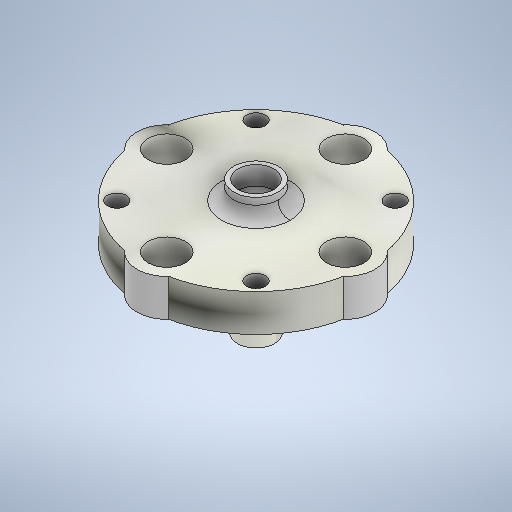
# Autodesk Inventor part: Redesign_Spinner
Saved by Autodesk Inventor 2025.1 (Build 291241000, 241)
## iProperties
Created: 2024-12-23
Part Number: Redesign_Spinner
Material: Generic
Document SubType Name: Modeling
Designer: m_kni
Density: 1 g/cm^3
Appearance: Default
Author: m_kni
Autodesk Inventor part; units mm, degrees
ref_plane "YZ Plane" through (0, 0, 0) normal (1, 0, 0) x (0, 1, 0)
ref_plane "XZ Plane" through (0, 0, 0) normal (0, 1, 0) x (-1, 0, 0)
ref_plane "XY Plane" through (0, 0, 0) normal (0, 0, 1) x (1, 0, 0)
sketch "Sketch1" plane through (0, 0, 0) normal (0, 1, 0) x (-1, 0, 0)
  circle A0 centre (0, 0) radius 2.5
  dimension "d0" = 5
  constraints: 1 centre point, 1 coincident
  measures "d0" diameter of A0
extrude "Extrusion1" add sketch "Sketch1" along normal blind 10.4
sketch "Sketch2" plane through (0, 10.4, 0) normal (0, 1, 0) x (1, 0, 0)
  circle A0 centre (0, 0) radius 12
  circle A1 centre (-12, 0) radius 1.5
  circle A2 centre (-12, 0) radius 2.5
  circle A3 centre (0, -12) radius 1.5
  circle A4 centre (0, -12) radius 2.5
  circle A5 centre (12, 0) radius 1.5
  circle A6 centre (12, 0) radius 2.5
  circle A7 centre (0, 12) radius 1.5
  circle A8 centre (0, 12) radius 2.5
  circle A9 centre (0, 0) radius 14.9832
  circle A10 centre (12, 0) radius 4
  circle A11 centre (0, -12) radius 4
  circle A12 centre (-12, 0) radius 4
  circle A13 centre (0, 12) radius 4
  point P0 (2.9628, -14.6873)
  point P1 (-2.9628, -14.6873)
  point P2 (-14.6873, -2.9628)
  point P3 (-14.6873, 2.9628)
  point P4 (-2.9628, 14.6873)
  point P5 (2.9628, 14.6873)
  point P6 (14.6873, 2.9628)
  point P7 (14.6873, -2.9628)
  dimension "d3" = 24
  dimension "d4" = 3
  dimension "d5" = 5
  dimension "d8" = 360
  dimension "d22" = 8
  dimension "d23" = 8
  dimension "d24" = 8
  dimension "d25" = 8
  constraints: 14 centre point, 6 coincident, 2 point on circle, 17 other
  measures "d3" diameter of A0
  measures "d4" diameter of A1
  measures "d5" diameter of A2
  measures "d22" diameter of A10
  measures "d23" diameter of A11
  measures "d24" diameter of A12
  measures "d25" diameter of A13
extrude "Extrusion2" add sketch "Sketch2" along normal blind 5 contours A6 A0 A10 | A0 A10 A9 A6 | A10 A0 A11 A12 A13 | A0 A13 A9 A10 | A10 A9 A11 A0 | A13 A0 A8 | A0 A8 A13 A9 | A10 A9 | A11 A9 A0 A4 | A0 A4 A11 | A0 A12 A9 A13 | A9 A13 | A11 A9 A12 A0 | A11 A9 | A12 A0 A2 | A0 A2 A12 A9 | A9 A12
fillet "Fillet1" radius 3.175 1 edges at (2.5, 10.4, 0)
sketch "Sketch3" plane through (0, 15.4, 0) normal (0, 1, 0) x (1, 0, 0)
  circle A0 centre (0, 0) radius 2.5 projected
  circle A1 centre (0, 0) radius 1.05
  dimension "d13" = 2.1
  constraints: 1 centre point, 1 coincident
  measures "d13" diameter of A1
extrude "Extrusion3" cut sketch "Sketch3" against normal blind 18.3375 contours A1
sketch "Sketch5" plane through (0, 0, 0) normal (0, -1, 0) x (1, 0, 0)
  circle A0 centre (0, 0) radius 1.05 projected
  circle A1 centre (0, 0) radius 1.825
  dimension "d19" = 3.65
  constraints: 1 centre point, 1 coincident
  measures "d19" diameter of A1
extrude "Extrusion5" cut sketch "Sketch5" against normal blind 12.4
sketch "Sketch6" plane through (0, 15.4, 0) normal (0, 1, 0) x (1, 0, 0)
  circle A0 centre (0, 0) radius 2
  circle A1 centre (0, 0) radius 1.05
  circle A2 centre (0, 0) radius 2.4
  circle A3 centre (0, 0) radius 1.05 projected
  circle A4 centre (0, 0) radius 3
  dimension "d26" = 4
  dimension "d30" = 4.8
  dimension "d31" = 6
  constraints: 4 centre point, 4 coincident
  measures "d26" diameter of A0
  measures "d30" diameter of A2
  measures "d31" diameter of A4
extrude "Extrusion6" add sketch "Sketch6" along normal blind 2.5 contours A4
fillet "Fillet3" radius 1.5875 1 edges at (-3, 15.4, 0) curvature continuous yes
sketch "Sketch7" plane through (0, 15.4, 0) normal (0, 1, 0) x (1, 0, 0)
  arc A0 (-14.6873, -2.9628) -> (-2.9628, -14.6873) centre (0, 0) ccw projected
  line L0 (0, 0) -> (-10.5947, -10.5947)
  line L1 (0, 0) -> (14.9832, 0) construction
  line L2 (0, 0) -> (-14.6873, 0)
  circle A1 centre (-9.3573, -9.3573) radius 1.25
  circle A2 centre (9.3573, -9.3573) radius 1.25
  circle A3 centre (9.3573, 9.3573) radius 1.25
  circle A4 centre (-9.3573, 9.3573) radius 1.25
  dimension "d33" = 135
  dimension "d36" = 2.5
  dimension "d39" = 360
  constraints: 6 end point, 4 centre point, 2 horizontal, 1 equal length, 1 point on circle, 1 point on line, 9 other
  measures "d33" angle of L0 L1
  measures "d36" diameter of A1
extrude "Extrusion7" cut sketch "Sketch7" against normal blind 10
body "Solid1"
